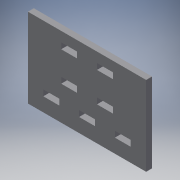
# Autodesk Inventor part: Side
Saved by Autodesk Inventor 2018 (Build 220112000, 112)
## iProperties
Created: 2017-10-30
Part Number: Side
Material: Polycarbonate, Clear
Document SubType Name: Modeling
Designer: xl0
Density: 1.2 g/cm^3
Appearance: Polycarbonate - Clear
Author: xl0
Autodesk Inventor part; units mm, degrees
ref_plane "YZ Plane" through (0, 0, 0) normal (1, 0, 0) x (0, 1, 0)
ref_plane "XZ Plane" through (0, 0, 0) normal (0, 1, 0) x (-1, 0, 0)
ref_plane "XY Plane" through (0, 0, 0) normal (0, 0, 1) x (1, 0, 0)
sketch "Sketch1" plane through (0, 0, 0) normal (0, 0, 1) x (1, 0, 0)
  line L0 (0, 8) -> (59.5, 8)
  line L1 (59.5, 8) -> (59.5, -32)
  line L2 (59.5, -32) -> (0, -32)
  line L3 (0, -32) -> (0, 8)
  line L4 (0, 0) -> (0, 3) construction
  line L5 (59.5, 0) -> (59.5, 3) construction
  line L6 (0, 3) -> (16.75, 3) construction
  line L7 (15.75, -25) -> (7.75, -25) projected
  line L8 (15.75, -25) -> (15.75, -22) projected
  line L9 (7.75, -22) -> (15.75, -22) projected
  line L10 (7.75, -25) -> (7.75, -22) projected
  line L11 (33.75, -25) -> (25.75, -25) projected
  line L12 (33.75, -25) -> (33.75, -22) projected
  line L13 (25.75, -22) -> (33.75, -22) projected
  line L14 (25.75, -25) -> (25.75, -22) projected
  line L15 (51.75, -25) -> (43.75, -25) projected
  line L16 (51.75, -25) -> (51.75, -22) projected
  line L17 (43.75, -22) -> (51.75, -22) projected
  line L18 (43.75, -25) -> (43.75, -22) projected
  line L19 (16.75, -15) -> (24.75, -15) projected
  line L20 (24.75, -15) -> (24.75, -12) projected
  line L21 (16.75, -12) -> (24.75, -12) projected
  line L22 (16.75, -15) -> (16.75, -12) projected
  line L23 (34.75, -15) -> (42.75, -15) projected
  line L24 (42.75, -15) -> (42.75, -12) projected
  line L25 (34.75, -12) -> (42.75, -12) projected
  line L26 (34.75, -15) -> (34.75, -12) projected
  line L27 (16.75, 0) -> (24.75, 0) projected
  line L28 (24.75, 0) -> (24.75, 3) projected
  line L29 (16.75, 3) -> (24.75, 3) projected
  line L30 (16.75, 0) -> (16.75, 3) projected
  line L31 (34.75, 0) -> (42.75, 0) projected
  line L32 (42.75, 0) -> (42.75, 3) projected
  line L33 (34.75, 3) -> (42.75, 3) projected
  line L34 (34.75, 0) -> (34.75, 3) projected
  dimension "d0" = 40
  dimension "d1" = 5
  constraints: 8 end point, 2 collinear, 2 parallel, 1 horizontal, 1 perpendicular
  measures "d0" distance between parallel lines of L2 L0
  measures "d1" distance between parallel lines of L0 L6
extrude "Extrusion1" add sketch "Sketch1" along normal blind 3
body "Solid1"
